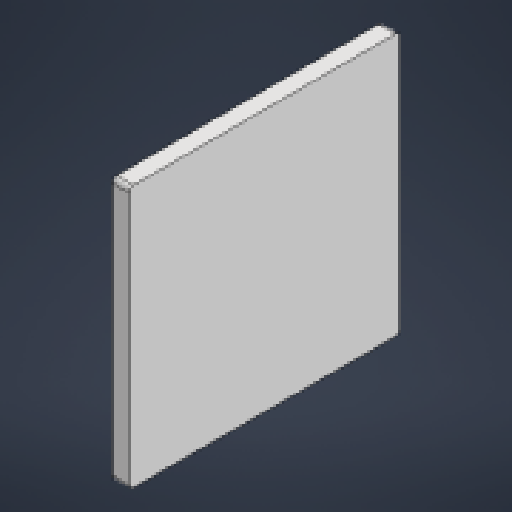
# Autodesk Inventor part: 3DPRINT,LIMIT_SWITCH,SPACER
Saved by Autodesk Inventor 2026.1 (Build 301233020, 233B)
## iProperties
Created: 2026-02-01
Part Number: 3DPRINT,LIMIT_SWITCH,SPACER
Material: ABS Plastic
Document SubType Name: Modeling
Designer: Owen L
Density: 1.06 g/cm^3
Appearance: Smooth - Black
Author: Owen L
Autodesk Inventor part; units mm, degrees
ref_plane "YZ Plane" through (0, 0, 0) normal (1, 0, 0) x (0, 1, 0)
ref_plane "XZ Plane" through (0, 0, 0) normal (0, 1, 0) x (-1, 0, 0)
ref_plane "XY Plane" through (0, 0, 0) normal (0, 0, 1) x (1, 0, 0)
sketch "Sketch1" plane through (0, 0, 0) normal (1, 0, 0) x (0, 1, 0)
  line L0 (15.5, -16) -> (-15.5, -16)
  line L1 (-15.5, -16) -> (-15.5, 16)
  line L2 (-15.5, 16) -> (15.5, 16)
  line L3 (15.5, 16) -> (15.5, -16)
  line L4 (15.5, -16) -> (-15.5, 16) construction
  line L5 (-15.5, -16) -> (15.5, 16) construction
  line L6 (-8.37, 8) -> (-8.37, -8) construction
  line L7 (-6.22, 8) -> (-6.22, -8)
  line L8 (-10.52, -8) -> (-10.52, 8)
  arc A0 (-6.22, 8) -> (-10.52, 8) centre (-8.37, 8) ccw
  arc A1 (-10.52, -8) -> (-6.22, -8) centre (-8.37, -8) ccw
  point P0 (0, 0)
  point P1 (-8.37, 0)
  dimension "d0" = 31
  dimension "d1" = 32
  dimension "d5" = 7.13
  dimension "d6" = 16
  dimension "d7" = 4.3
  constraints: 20 end point, 4 parallel, 4 point on circle, 4 tangent, 3 midpoint, 2 centre point, 1 horizontal, 1 horizontal alignment, 1 perpendicular
  measures "d0" distance of L1.end L2.end
  measures "d1" distance of L0.end L1.end
  measures "d5" distance between parallel lines of L1 L6
  measures "d6" distance of L6.start L6.end
  measures "d7" distance of L7.end L8.start
extrude "Extrusion1" add sketch "Sketch1" along normal blind 2
fillet "Fillet1" radius 0.5 4 edges at (1, 15.5, 16) (1, -15.5, 16) (1, -15.5, -16) (1, 15.5, -16)
body "Solid1"
